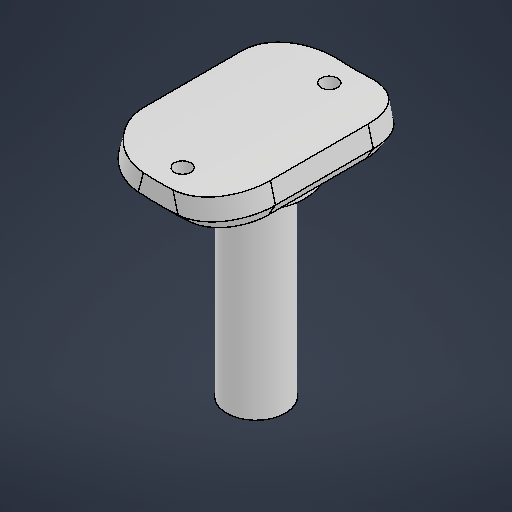
# Autodesk Inventor part: Mount_A
Saved by Autodesk Inventor 2026.1 (Build 301233000, 233)
## iProperties
Created: 2025-10-12
Part Number: Mount_A
Material: Generic
Document SubType Name: Modeling
Designer: 1char
Mass: 11.0226 g
Surface Area: 43.5808 cm^2
Volume: 11.0226 cm^3
Density: 1 g/cm^3
Appearance: Default
Author: 1char
Autodesk Inventor part; units mm, degrees
ref_plane "YZ Plane" through (0, 0, 0) normal (1, 0, 0) x (0, 1, 0)
ref_plane "XZ Plane" through (0, 0, 0) normal (0, 1, 0) x (-1, 0, 0)
ref_plane "XY Plane" through (0, 0, 0) normal (0, 0, 1) x (1, 0, 0)
sketch "Sketch1" plane through (0, 0, 0) normal (0, 0, 1) x (1, 0, 0)
  arc A0 (-12.941, 7.7037) -> (12.941, 7.7037) centre (0, 56) ccw
  arc A1 (-14.4939, 1.9082) -> (14.4939, 1.9082) centre (0, 56) ccw
  line L0 (-14.4939, 1.9082) -> (-12.941, 7.7037)
  line L1 (14.4939, 1.9082) -> (12.941, 7.7037)
  line L2 (0, -11.2) -> (0, 67.2) construction
  point P0 (0, 0)
  dimension "d0" = 6
  dimension "d1" = 50
  dimension "d2" = 30
  constraints: 5 point on circle, 4 end point, 3 point on line, 2 centre point, 1 concentric, 1 other
  measures "d0" distance of L1.start L1.end
  measures "d1" radius of A0
  measures "d2" angle of L1 L0
extrude "Extrusion1" add sketch "Sketch1" along normal mid plane 40
sketch "Sketch2" plane through (0, 0, 0) normal (0, 1, 0) x (-1, 0, 0)
  point P0 (0, 0)
  point P1 (0, -15)
  point P2 (0, 15)
  dimension "d5" = 15
  dimension "d6" = 15
  constraints: 2 vertical alignment
  measures "d5" distance of point (0, -15) point (0, 0)
  measures "d6" distance of point (0, 0) point (0, 15)
hole "Hole1" at (0, 0, -15) at (0, 0, 15) direction (0, 1, 0) diameter 3.4 end through all clearance for "Socket Head Cap Screw DIN EN ISO 4762" size "M3" standard "DIN"
sketch "Sketch4" plane through (0, 0, 0) normal (0, 1, 0) x (-1, 0, 0)
  circle A0 centre (0, 0) radius 10
  dimension "d20" = 20
  constraints: 1 centre point, 1 coincident
  measures "d20" diameter of A0
extrude "Extrusion3" add sketch "Sketch4" along normal up to surface
extrude "Extrusion4" add sketch "Sketch4" against normal blind 2
fillet "Fillet2" radius 10 4 edges at (-13.7174, 4.8059, -20) (13.7174, 4.8059, -20) (13.7174, 4.8059, 20) (-13.7174, 4.8059, 20)
sketch "Sketch6" plane through (0, -2, 0) normal (0, -1, 0) x (1, 0, 0)
  circle A0 centre (0, 0) radius 6
  dimension "d27" = 12
  constraints: 1 centre point, 1 coincident
  measures "d27" diameter of A0
extrude "Extrusion5" add sketch "Sketch6" along normal blind 40
chamfer "Chamfer1" distance 2 angle 45 4 edges at (14.4939, 1.9082, 0) (0, 0, -20) (-14.4939, 1.9082, 0) (0, 0, 20)
equation "\"d6\" = d5"
body "Solid1"
